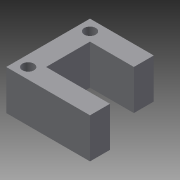
# Autodesk Inventor part: OfflineBowdenExtruder
Saved by Autodesk Inventor 2015 SP1 (Build 190203100, 203)
## iProperties
Created: 2015-04-29
Part Number: OfflineBowdenExtruder
Material: Generic
Document SubType Name: Modeling
Designer: Jack
Density: 1 g/cm^3
Appearance: Default
Author: Jack
Autodesk Inventor part; units mm, degrees
ref_plane "YZ Plane" through (0, 0, 0) normal (1, 0, 0) x (0, 1, 0)
ref_plane "XZ Plane" through (0, 0, 0) normal (0, 1, 0) x (-1, 0, 0)
ref_plane "XY Plane" through (0, 0, 0) normal (0, 0, 1) x (1, 0, 0)
sketch "Sketch1" plane through (0, 0, 0) normal (0, 0, 1) x (1, 0, 0)
  line L0 (0, 0) -> (42, 0)
  line L1 (0, 0) -> (0, 42)
  line L2 (0, 42) -> (32, 42)
  line L3 (32, 42) -> (32, 32)
  line L4 (32, 32) -> (10, 32)
  line L5 (10, 32) -> (10, 10)
  line L6 (10, 10) -> (42, 10)
  line L7 (42, 10) -> (42, 0)
  dimension "d0" = 42
  dimension "d1" = 42
  dimension "d2" = 32
  dimension "d3" = 10
  dimension "d5" = 10
  dimension "d6" = 10
  constraints: 16 end point, 5 perpendicular, 2 vertical, 1 horizontal
  measures "d0" distance of L0.start L0.end
  measures "d1" distance of L0.start L1.end
  measures "d2" distance of L1.end L2.end
  measures "d3" distance of L2.end L3.end
  measures "d5" distance between parallel lines of L0 L6
  measures "d6" distance between parallel lines of L1 L5
extrude "Extrusion1" add sketch "Sketch1" along normal blind 20
sketch "Sketch2" plane through (0, 0, 20) normal (0, 0, 1) x (1, 0, 0)
  line L0 (32, 42) -> (0, 42) projected
  line L1 (0, 42) -> (0, 0) projected
  point P0 (5.5, 36.5)
  point P1 (5.5, 5.5)
  dimension "d9" = 31
  dimension "d11" = 5.5
  dimension "d13" = 5.5
  constraints: 1 vertical alignment
  measures "d9" distance of point (5.5, 5.5) point (5.5, 36.5)
  measures "d11" distance from line of L0 point (5.5, 36.5)
  measures "d13" distance from line of L1 point (5.5, 5.5)
hole "Hole1" at (5.5, 36.5, 20) at (5.5, 5.5, 20) direction (0, 0, -1) diameter 3.5 end through all counterbore diameter 5.8 counterbore depth 15
body "Solid1"
